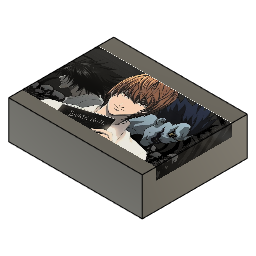
The_Shinigami_bot (Autodesk Fusion 360 archive; units mm, degrees)
design "battery"
Autodesk Fusion 360 part; units mm, degrees
sketch "Sketch1" plane through (0, 0, 0) normal (0, 0, 1) x (1, 0, 0)
  line L0 (-26.6654, -18.678) -> (43.3346, -18.678)
  line L1 (43.3346, -18.678) -> (43.3346, 36.322)
  line L2 (43.3346, 36.322) -> (-26.6654, 36.322)
  line L3 (-26.6654, 36.322) -> (-26.6654, -18.678)
  dimension "d1" = 70
  dimension "d2" = 55
  constraint horizontal L0
  constraint vertical L1
  constraint horizontal L2
  constraint vertical L3
  measures "d1" distance of L0.start L0.end
  measures "d2" distance of L0.start L2.end
extrude "Extrude1" add sketch "Sketch1" along normal blind 20

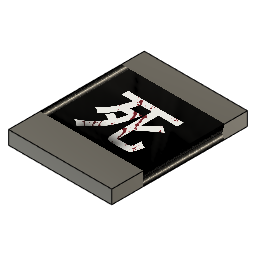
design "solder board"
Autodesk Fusion 360 part; units mm, degrees
sketch "Sketch1" plane through (0, 0, 0) normal (0, 0, 1) x (1, 0, 0)
  line L0 (-44.1146, 29.4917) -> (31.8854, 29.4917)
  line L1 (31.8854, 29.4917) -> (31.8854, -70.5083)
  line L2 (31.8854, -70.5083) -> (-44.1146, -70.5083)
  line L3 (-44.1146, -70.5083) -> (-44.1146, 29.4917)
  dimension "d1" = 76
  dimension "d2" = 100
  constraint horizontal L0
  constraint vertical L1
  constraint horizontal L2
  constraint vertical L3
  measures "d1" distance of L0.start L0.end
  measures "d2" distance of L0.start L2.end
extrude "Extrude1" add sketch "Sketch1" along normal blind 10

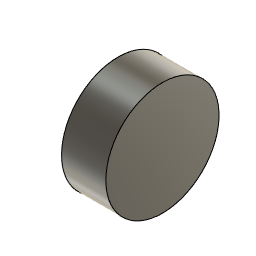
design "wheel"
Autodesk Fusion 360 part; units mm, degrees
sketch "Sketch1" plane through (0, 0, 0) normal (1, 0, 0) x (0, 1, 0)
  circle A0 centre (0, 0) radius 57.5
  dimension "d2" = 115
  constraint coincident A0.centre origin
  measures "d2" diameter of A0
extrude "Extrude1" add sketch "Sketch1" along normal blind 45
ref_plane "WorkPlane2" through (-25, 0, 0) normal (1, 0, 0) x (0, 1, 0)
sketch "Sketch2" plane through (-25, 0, 0) normal (1, 0, 0) x (0, 1, 0)
  circle A0 centre (0, 0) radius 20
  dimension "d7" = 40
  constraint coincident A0.centre origin
  measures "d7" diameter of A0
extrude "Extrude2" add sketch "Sketch2" along normal up to surface (25 mm away)
